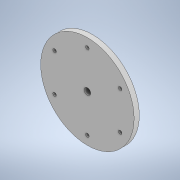
# Autodesk Inventor part: disco
Saved by Autodesk Inventor 2020 (Build 240168000, 168)
## iProperties
Created: 2021-02-16
Part Number: disco
Material: Generic
Document SubType Name: Modeling
Designer: vinig
Density: 1 g/cm^3
Appearance: Default
Author: vinig
Autodesk Inventor part; units mm, degrees
ref_plane "YZ Plane" through (0, 0, 0) normal (1, 0, 0) x (0, 1, 0)
ref_plane "XZ Plane" through (0, 0, 0) normal (0, 1, 0) x (-1, 0, 0)
ref_plane "XY Plane" through (0, 0, 0) normal (0, 0, 1) x (1, 0, 0)
sketch "Sketch1" plane through (0, 0, 0) normal (0, 0, 1) x (1, 0, 0)
  circle A0 centre (0, 0) radius 90.35
  circle A1 centre (0, 0) radius 6.35
  circle A2 centre (0, 73.25) radius 3.4
  circle A3 centre (-63.4364, 36.625) radius 3.4
  circle A4 centre (-63.4364, -36.625) radius 3.4
  line L0 (0, 0) -> (35.2961, 61.1346)
  circle A5 centre (63.4364, 36.625) radius 3.4
  circle A6 centre (63.4364, -36.625) radius 3.4
  circle A7 centre (0, -73.25) radius 3.4
  line L1 (0, 0) -> (0, 73.25)
  dimension "d1" = 180.7
  dimension "d2" = 12.7
  dimension "d3" = 6.8
  dimension "d5" = 73.25
  dimension "d6" = 6.8
  dimension "d7" = 73.25
  dimension "d8" = 60
  dimension "d10" = 6.8
  dimension "d11" = 73.25
  dimension "d12" = 60
  dimension "d13" = 30
  constraints: 8 centre point, 4 end point, 3 symmetric about line, 2 coincident, 1 vertical, 3 other
  measures "d1" diameter of A0
  measures "d2" diameter of A1
  measures "d3" diameter of A2
  measures "d5" distance of point (0, 0) L1.end
  measures "d6" diameter of A3
  measures "d7" distance of point (0, 0) A3.centre
  measures "d10" diameter of A4
  measures "d11" distance of point (0, 0) A4.centre
extrude "Extrusion1" add sketch "Sketch1" along normal blind 10
body "Solid1"
